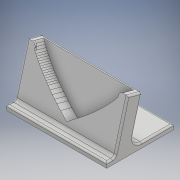
# Autodesk Inventor part: Supporto3
Saved by Autodesk Inventor 2018 (Build 220112000, 112)
## iProperties
Created: 2020-01-19
Part Number: Supporto3
Material: Generic
Document SubType Name: Modeling
Designer: Lorenzo Spadaro
Density: 1 g/cm^3
Appearance: Default
Author: Lorenzo Spadaro
Autodesk Inventor part; units mm, degrees
ref_plane "YZ Plane" through (0, 0, 0) normal (1, 0, 0) x (0, 1, 0)
ref_plane "XZ Plane" through (0, 0, 0) normal (0, 1, 0) x (-1, 0, 0)
ref_plane "XY Plane" through (0, 0, 0) normal (0, 0, 1) x (1, 0, 0)
sketch "Sketch1" plane through (0, 0, 0) normal (0, 0, 1) x (1, 0, 0)
  line L0 (-30, -20) -> (30, -20)
  line L1 (30, -20) -> (30, 20)
  line L2 (30, 20) -> (-30, 20)
  line L3 (-30, 20) -> (-30, -20)
  line L4 (-30, -20) -> (30, 20) construction
  line L5 (30, -20) -> (-30, 20) construction
  point P0 (0, 0)
  dimension "d0" = 60
  dimension "d1" = 40
  constraints: 12 end point, 2 midpoint, 2 parallel, 1 horizontal, 1 perpendicular
  measures "d0" distance of L2.end L1.end
  measures "d1" distance of L1.end L0.end
extrude "Extrusion1" add sketch "Sketch1" along normal blind 3
sketch "Sketch2" plane through (-30, -20, 0) normal (-1, 0, 0) x (0, 0, 1)
  line L0 (0, 0) -> (0, 40) projected
  line L1 (3, 40) -> (0, 40)
  line L2 (0, 40) -> (0, 0)
  line L3 (0, 0) -> (3, 0)
  line L4 (0, 40) -> (0, 20)
  line L5 (3, 40) -> (3, 5)
  line L6 (3, 5) -> (0, 5)
  line L7 (3, 0) -> (3, 40) projected
  line L8 (3, 5) -> (3, 0)
  line L9 (3, 5) -> (3, 12.6)
  line L10 (3, 12.6) -> (6, 12.6) construction
  line L11 (6.1624, 5.8474) -> (3, 5)
  line L12 (6.1624, 5.8474) -> (4.3531, 12.6)
  line L13 (6.1624, 5.8474) -> (13.1533, 5.8474) construction
  line L14 (4.3531, 12.6) -> (3, 12.6)
  dimension "d5" = 35
  dimension "d19" = 105
  dimension "d26" = 7.6
  dimension "d27" = 105
  constraints: 26 end point, 3 collinear, 3 horizontal, 3 point on line, 2 perpendicular, 1 equal length, 1 vertical
  measures "d5" distance of L1.start L5.end
  measures "d19" angle of L13 L12
  measures "d26" distance from line of L5.end L10
  measures "d27" angle of L7 L11
extrude "Extrusion2" add sketch "Sketch2" against normal blind 60 contours L5 L14 L12 L11
sketch "Sketch3" plane through (-30, -15, 3) normal (0, -0.9659258, 0.258819) x (1, 0, 0)
  line L0 (0, 3.274) -> (60, 3.274) projected
  line L1 (12.5923, 64.1788) -> (12.9587, 64.2079)
  line L2 (12.9587, 64.2079) -> (15.1774, 64.2905)
  line L3 (15.1774, 64.2905) -> (16.662, 64.2406)
  line L4 (16.662, 64.2406) -> (17.7697, 64.1374)
  line L5 (17.7697, 64.1374) -> (18.867, 63.9707)
  line L6 (18.867, 63.9707) -> (19.5902, 63.8211)
  line L7 (19.5902, 63.8211) -> (20.305, 63.6386)
  line L8 (20.305, 63.6386) -> (21.0099, 63.4212)
  line L9 (21.0099, 63.4212) -> (21.7034, 63.1671)
  line L10 (21.7034, 63.1671) -> (22.3839, 62.8743)
  line L11 (22.3839, 62.8743) -> (23.0499, 62.541)
  line L12 (23.0499, 62.541) -> (23.3315, 62.391)
  line L13 (23.3315, 62.391) -> (24.1498, 61.9043)
  line L14 (24.1498, 61.9043) -> (25.1851, 61.1786)
  line L15 (25.1851, 61.1786) -> (26.4008, 60.1685)
  line L16 (26.4008, 60.1685) -> (29.8855, 56.4868)
  line L17 (29.8855, 56.4868) -> (33.7036, 60.5226)
  line L18 (33.7036, 60.5226) -> (35.0763, 61.6118)
  line L19 (35.0763, 61.6118) -> (36.0566, 62.2564)
  line L20 (36.0566, 62.2564) -> (36.399, 62.4589)
  line L21 (36.399, 62.4589) -> (36.7462, 62.6497)
  line L22 (36.7462, 62.6497) -> (37.0981, 62.8293)
  line L23 (37.0981, 62.8293) -> (37.4543, 62.9976)
  line L24 (37.4543, 62.9976) -> (37.8145, 63.1551)
  line L25 (37.8145, 63.1551) -> (38.5466, 63.4386)
  line L26 (38.5466, 63.4386) -> (39.2924, 63.6816)
  line L27 (39.2924, 63.6816) -> (40.05, 63.8862)
  line L28 (40.05, 63.8862) -> (40.8179, 64.0543)
  line L29 (40.8179, 64.0543) -> (41.5938, 64.1878)
  line L30 (41.5938, 64.1878) -> (42.3761, 64.2888)
  line L31 (42.3761, 64.2888) -> (43.5574, 64.3837)
  line L32 (43.5574, 64.3837) -> (45.1374, 64.4148)
  line L33 (45.1374, 64.4148) -> (47.0997, 64.3228)
  line L34 (47.0997, 64.3228) -> (47.4823, 64.2889)
  line L35 (47.4823, 64.2889) -> (47.8629, 64.2434)
  line L36 (47.8629, 64.2434) -> (48.2415, 64.1869)
  line L37 (48.2415, 64.1869) -> (48.9917, 64.041)
  line L38 (48.9917, 64.041) -> (49.7314, 63.8526)
  line L39 (49.7314, 63.8526) -> (50.4592, 63.6235)
  line L40 (50.4592, 63.6235) -> (51.1737, 63.3553)
  line L41 (51.1737, 63.3553) -> (51.8735, 63.0494)
  line L42 (51.8735, 63.0494) -> (52.5571, 62.7077)
  line L43 (52.5571, 62.7077) -> (53.2231, 62.3315)
  line L44 (53.2231, 62.3315) -> (53.8701, 61.9227)
  line L45 (53.8701, 61.9227) -> (54.4966, 61.4826)
  line L46 (54.4966, 61.4826) -> (55.1012, 61.0131)
  line L47 (55.1012, 61.0131) -> (55.6826, 60.5156)
  line L48 (55.6826, 60.5156) -> (56.2392, 59.9919)
  line L49 (56.2392, 59.9919) -> (56.7697, 59.4434)
  line L50 (56.7697, 59.4434) -> (57.0867, 59.0974)
  line L51 (57.0867, 59.0974) -> (57.3931, 58.7432)
  line L52 (57.3931, 58.7432) -> (57.6888, 58.3813)
  line L53 (57.6888, 58.3813) -> (57.9739, 58.0118)
  line L54 (57.9739, 58.0118) -> (58.2485, 57.6351)
  line L55 (58.2485, 57.6351) -> (58.5128, 57.2515)
  line L56 (58.5128, 57.2515) -> (58.7666, 56.8611)
  line L57 (58.7666, 56.8611) -> (59.0103, 56.4645)
  line L58 (59.0103, 56.4645) -> (59.2438, 56.0618)
  line L59 (59.2438, 56.0618) -> (59.4672, 55.6533)
  line L60 (59.4672, 55.6533) -> (59.6807, 55.2393)
  line L61 (59.6807, 55.2393) -> (60.078, 54.3962)
  line L62 (60.078, 54.3962) -> (60.4362, 53.5346)
  line L63 (60.4362, 53.5346) -> (60.7561, 52.657)
  line L64 (60.7561, 52.657) -> (61.0385, 51.7657)
  line L65 (61.0385, 51.7657) -> (61.2838, 50.8632)
  line L66 (61.2838, 50.8632) -> (61.4928, 49.9515)
  line L67 (61.4928, 49.9515) -> (61.6662, 49.0333)
  line L68 (61.6662, 49.0333) -> (61.8045, 48.1108)
  line L69 (61.8045, 48.1108) -> (61.9085, 47.1863)
  line L70 (61.9085, 47.1863) -> (61.9254, 43.1345)
  line L71 (61.9254, 43.1345) -> (61.8677, 42.5497)
  line L72 (61.8677, 42.5497) -> (61.7957, 41.9643)
  line L73 (61.7957, 41.9643) -> (61.7102, 41.3817)
  line L74 (61.7102, 41.3817) -> (61.6114, 40.802)
  line L75 (61.6114, 40.802) -> (61.4997, 40.2253)
  line L76 (61.4997, 40.2253) -> (61.3754, 39.6515)
  line L77 (61.3754, 39.6515) -> (61.2388, 39.0809)
  line L78 (61.2388, 39.0809) -> (61.0903, 38.5134)
  line L79 (61.0903, 38.5134) -> (60.9299, 37.9491)
  line L80 (60.9299, 37.9491) -> (60.7584, 37.3881)
  line L81 (60.7584, 37.3881) -> (60.5757, 36.8305)
  line L82 (60.5757, 36.8305) -> (60.1784, 35.7255)
  line L83 (60.1784, 35.7255) -> (59.7408, 34.6348)
  line L84 (59.7408, 34.6348) -> (59.2652, 33.559)
  line L85 (59.2652, 33.559) -> (58.7541, 32.4985)
  line L86 (58.7541, 32.4985) -> (58.2101, 31.4539)
  line L87 (58.2101, 31.4539) -> (57.6357, 30.4258)
  line L88 (57.6357, 30.4258) -> (56.7225, 28.9157)
  line L89 (56.7225, 28.9157) -> (55.7548, 27.4457)
  line L90 (55.7548, 27.4457) -> (55.2622, 26.7446)
  line L91 (55.2622, 26.7446) -> (54.7597, 26.0515)
  line L92 (54.7597, 26.0515) -> (54.2477, 25.3661)
  line L93 (54.2477, 25.3661) -> (53.7265, 24.6882)
  line L94 (53.7265, 24.6882) -> (53.1963, 24.0177)
  line L95 (53.1963, 24.0177) -> (52.1103, 22.6982)
  line L96 (52.1103, 22.6982) -> (50.9918, 21.4064)
  line L97 (50.9918, 21.4064) -> (49.8431, 20.141)
  line L98 (49.8431, 20.141) -> (48.6664, 18.9008)
  line L99 (48.6664, 18.9008) -> (47.4641, 17.6844)
  line L100 (47.4641, 17.6844) -> (45.6174, 15.902)
  line L101 (45.6174, 15.902) -> (43.7254, 14.166)
  line L102 (43.7254, 14.166) -> (40.4923, 11.3651)
  line L103 (40.4923, 11.3651) -> (38.5167, 9.7327)
  line L104 (38.5167, 9.7327) -> (30.1085, 3.3998)
  line L105 (30.1085, 3.3998) -> (25.6132, 6.6417)
  line L106 (25.6132, 6.6417) -> (22.9564, 8.65)
  line L107 (22.9564, 8.65) -> (21.2085, 10.0198)
  line L108 (21.2085, 10.0198) -> (19.4827, 11.4167)
  line L109 (19.4827, 11.4167) -> (17.7822, 12.8431)
  line L110 (17.7822, 12.8431) -> (16.1101, 14.3009)
  line L111 (16.1101, 14.3009) -> (15.2856, 15.0423)
  line L112 (15.2856, 15.0423) -> (14.4694, 15.7925)
  line L113 (14.4694, 15.7925) -> (13.6619, 16.5517)
  line L114 (13.6619, 16.5517) -> (12.8633, 17.32)
  line L115 (12.8633, 17.32) -> (12.0742, 18.0979)
  line L116 (12.0742, 18.0979) -> (11.2948, 18.8857)
  line L117 (11.2948, 18.8857) -> (10.5256, 19.6835)
  line L118 (10.5256, 19.6835) -> (9.767, 20.4915)
  line L119 (9.767, 20.4915) -> (9.0194, 21.3102)
  line L120 (9.0194, 21.3102) -> (8.2831, 22.1398)
  line L121 (8.2831, 22.1398) -> (7.5585, 22.9805)
  line L122 (7.5585, 22.9805) -> (6.846, 23.8326)
  line L123 (6.846, 23.8326) -> (6.1461, 24.6965)
  line L124 (6.1461, 24.6965) -> (5.2953, 25.8036)
  line L125 (5.2953, 25.8036) -> (4.4707, 26.9361)
  line L126 (4.4707, 26.9361) -> (3.6761, 28.0931)
  line L127 (3.6761, 28.0931) -> (2.9153, 29.274)
  line L128 (2.9153, 29.274) -> (2.5487, 29.8734)
  line L129 (2.5487, 29.8734) -> (2.1921, 30.4785)
  line L130 (2.1921, 30.4785) -> (1.8457, 31.0893)
  line L131 (1.8457, 31.0893) -> (1.5103, 31.7058)
  line L132 (1.5103, 31.7058) -> (1.1861, 32.3279)
  line L133 (1.1861, 32.3279) -> (0.8737, 32.9555)
  line L134 (0.8737, 32.9555) -> (0.5736, 33.5885)
  line L135 (0.5736, 33.5885) -> (0.2862, 34.2269)
  line L136 (0.2862, 34.2269) -> (0.0121, 34.8706)
  line L137 (0.0121, 34.8706) -> (-0.2484, 35.5196)
  line L138 (-0.2484, 35.5196) -> (-0.4948, 36.1737)
  line L139 (-0.4948, 36.1737) -> (-0.7264, 36.8329)
  line L140 (-0.7264, 36.8329) -> (-0.943, 37.4971)
  line L141 (-0.943, 37.4971) -> (-1.144, 38.1663)
  line L142 (-1.144, 38.1663) -> (-1.3288, 38.8403)
  line L143 (-1.3288, 38.8403) -> (-1.4972, 39.5191)
  line L144 (-1.4972, 39.5191) -> (-1.6485, 40.2028)
  line L145 (-1.6485, 40.2028) -> (-1.7824, 40.891)
  line L146 (-1.7824, 40.891) -> (-1.8982, 41.584)
  line L147 (-1.8982, 41.584) -> (-1.9957, 42.2814)
  line L148 (-1.9957, 42.2814) -> (-2.0741, 42.9832)
  line L149 (-2.0741, 42.9832) -> (-2.0895, 46.6765)
  line L150 (-2.0895, 46.6765) -> (-1.9617, 47.905)
  line L151 (-1.9617, 47.905) -> (-1.776, 49.1288)
  line L152 (-1.776, 49.1288) -> (-1.5304, 50.3428)
  line L153 (-1.5304, 50.3428) -> (-1.2225, 51.5419)
  line L154 (-1.2225, 51.5419) -> (-0.8502, 52.7214)
  line L155 (-0.8502, 52.7214) -> (-0.5652, 53.4944)
  line L156 (-0.5652, 53.4944) -> (-0.2499, 54.2551)
  line L157 (-0.2499, 54.2551) -> (0.0962, 55.0017)
  line L158 (0.0962, 55.0017) -> (0.474, 55.7332)
  line L159 (0.474, 55.7332) -> (0.8839, 56.4478)
  line L160 (0.8839, 56.4478) -> (1.3267, 57.1442)
  line L161 (1.3267, 57.1442) -> (1.803, 57.8209)
  line L162 (1.803, 57.8209) -> (2.0705, 58.1743)
  line L163 (2.0705, 58.1743) -> (2.3475, 58.5211)
  line L164 (2.3475, 58.5211) -> (2.634, 58.8609)
  line L165 (2.634, 58.8609) -> (2.9297, 59.1934)
  line L166 (2.9297, 59.1934) -> (3.2344, 59.5184)
  line L167 (3.2344, 59.5184) -> (3.5476, 59.8355)
  line L168 (3.5476, 59.8355) -> (3.8693, 60.1443)
  line L169 (3.8693, 60.1443) -> (4.1992, 60.4445)
  line L170 (4.1992, 60.4445) -> (4.5371, 60.7359)
  line L171 (4.5371, 60.7359) -> (4.8827, 61.0179)
  line L172 (4.8827, 61.0179) -> (5.2358, 61.2904)
  line L173 (5.2358, 61.2904) -> (5.596, 61.5529)
  line L174 (5.596, 61.5529) -> (5.9633, 61.8052)
  line L175 (5.9633, 61.8052) -> (6.3373, 62.047)
  line L176 (6.3373, 62.047) -> (6.7178, 62.2778)
  line L177 (6.7178, 62.2778) -> (7.1046, 62.4974)
  line L178 (7.1046, 62.4974) -> (7.4974, 62.7054)
  line L179 (7.4974, 62.7054) -> (7.896, 62.9016)
  line L180 (7.896, 62.9016) -> (8.3001, 63.0854)
  line L181 (8.3001, 63.0854) -> (8.7095, 63.2568)
  line L182 (8.7095, 63.2568) -> (9.1239, 63.4152)
  line L183 (9.1239, 63.4152) -> (9.5432, 63.5605)
  line L184 (9.5432, 63.5605) -> (9.967, 63.6921)
  line L185 (9.967, 63.6921) -> (10.3952, 63.8099)
  line L186 (10.3952, 63.8099) -> (10.8274, 63.9135)
  line L187 (10.8274, 63.9135) -> (11.2635, 64.0025)
  line L188 (11.2635, 64.0025) -> (11.7031, 64.0766)
  line L189 (11.7031, 64.0766) -> (12.1462, 64.1355)
  line L190 (12.1462, 64.1355) -> (12.5923, 64.1788)
  line L191 (0, 0) -> (0, 3.274) projected
  line L192 (0, 3.274) -> (0, 29.274)
  line L193 (0, 29.274) -> (2.9153, 29.274)
  line L194 (60, 3.274) -> (60, 0) projected
  line L195 (60, 3.274) -> (60, 29.274)
  line L196 (60, 29.274) -> (56.9392, 29.274)
  point P0 (30, 0.9845)
  dimension "d0" = 60
  dimension "d15" = 26
  dimension "d16" = 26
  constraints: 388 end point, 4 perpendicular, 2 point on line, 1 horizontal, 1 parallel, 1 vertical
  measures "d15" distance of L0.start L192.end
  measures "d16" distance of L0.end L195.end
extrude "Extrusion3" add sketch "Sketch3" against normal blind 7 contours L192 L193 L127 L126 L125 L124 L123 L122 L121 L120 L119 L118 L117 L116 L115 L114 L113 L112 L111 L110 L109 L108 L107 L106 L105 L104 L103 L102 L101 L100 L99 L98 L97 L96 L95 L94 L93 L92 L91 L90 L89 L88 L196 L195 L0
sketch "Sketch4" plane through (26.9392, -7.4233, 31.2765) normal (0, 0.258819, 0.9659258) x (1, 0, 0)
  line L0 (3.0608, 7) -> (3.0608, 7) projected
  line L1 (-56.9392, 7) -> (-56.9392, 7) projected
  line L2 (-56.9392, 7) -> (3.0608, 7)
  line L3 (-56.9392, 5.4078) -> (3.0608, 5.4078) projected
  line L4 (-56.9392, 7) -> (-56.9392, 9)
  line L5 (-56.9392, 34.5839) -> (-56.9392, -4.0532) projected
  line L6 (-56.9392, 9) -> (3.0608, 9)
  line L7 (3.0608, 9) -> (3.0608, 7)
  line L8 (3.0608, -4.0532) -> (3.0608, 34.5839) projected
  point P0 (-26.9392, 15.2653)
  point P1 (-56.9392, 7.341)
  point P2 (3.0608, 7.341)
  dimension "d23" = 2
  constraints: 8 end point, 1 collinear, 1 perpendicular, 1 point on line
  measures "d23" distance of L1.start L4.end
extrude "Extrusion5" add sketch "Sketch4" against normal blind 28 contours L4 L6 L7 L2
sketch "Sketch5" plane through (-30, -15, 3) normal (0, -0.9659258, 0.258819) x (1, 0, 0)
  line L0 (60, 29.274) -> (0, 29.274) projected
  line L1 (60, 29.274) -> (55, 29.274)
  line L2 (55, 29.274) -> (55, 26.274)
  line L3 (55, 26.274) -> (60, 26.274)
  line L4 (60, 0) -> (60, 29.274) projected
  line L5 (60, 29.274) -> (60, 26.274)
  line L6 (0, 0) -> (0, 29.274) projected
  line L7 (0, 29.274) -> (0, 26.274)
  line L8 (0, 26.274) -> (5, 26.274)
  line L9 (5, 26.274) -> (5, 29.274)
  point P0 (30, 0.9845)
  dimension "d28" = 5
  dimension "d29" = 3
  dimension "d30" = 3
  dimension "d31" = 5
  constraints: 14 end point, 5 point on line, 2 perpendicular, 1 collinear, 1 vertical
  measures "d28" distance of L0.start L1.end
  measures "d29" distance of L1.end L2.end
  measures "d30" distance of L0.end L7.end
  measures "d31" distance of L7.end L8.end
extrude "Extrusion6" add sketch "Sketch5" against normal blind 1
fillet "Fillet1" radius 2 6 edges at (-25, -6.9404, 31.1471) (-25, -7.7168, 28.2493) (-25.0472, -7.7168, 28.2493) (25, -6.9404, 31.1471) (25, -7.6886, 28.3546) (0, -15, 3)
fillet "Fillet2" radius 5 1 edges at (0, -5.6825, 3)
fillet "Fillet3" radius 1 17 edges at (-30, -1.363, 19.1206) (-30, -3.1331, 4.9562) (-30, 10.4168, 3) (30, 10.4168, 3) (30, -1.363, 19.1206) (30, -3.1331, 4.9562) (0, 1.27, 28.9471) (-30, -3.0767, 30.1118) (30, -3.0767, 30.1118) (-30, -15.3171, 3.4133) (-30, -18.2673, 3) (-30, -11.0131, 17.8794) (30, -15.3171, 3.4133) (30, -18.2673, 3) (30, -11.0131, 17.8794) (0, -20, 3) (0, 20, 3)
body "Solid1"
